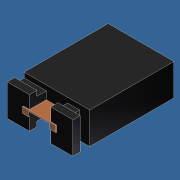
# Autodesk Inventor part: 2009_CTS_CopperPost2
Saved by Autodesk Inventor 2012 (Build 160160000, 160)
## iProperties
Company: Team 801
Created: 2009-01-31
Part Number: 2009_CTS_CopperPost2
Document SubType Name: Modeling
Designer: Jeffrey M
Density: 1 g/cm^3
Material: Default
Title: 2009_CTS_CopperPost2
Author: Jeffrey M
Autodesk Inventor part; units mm, degrees
ref_plane "YZ Plane" through (0, 0, 0) normal (1, 0, 0) x (0, 1, 0)
ref_plane "XZ Plane" through (0, 0, 0) normal (0, 1, 0) x (-1, 0, 0)
ref_plane "XY Plane" through (0, 0, 0) normal (0, 0, 1) x (1, 0, 0)
sketch "Sketch1" plane through (0, 0, 0) normal (0, 0, 1) x (1, 0, 0)
  line L0 (-37.8857, 18.2857) -> (-32.9327, 18.2857)
  line L1 (-32.9327, 18.2857) -> (-32.9327, 15.8981)
  line L2 (-32.9327, 15.8981) -> (-37.8857, 15.8981)
  line L3 (-37.8857, 15.8981) -> (-37.8857, 18.2857)
  dimension "d0" = 4.953
  dimension "d1" = 2.3876
  constraints: 8 end point, 2 parallel, 1 horizontal, 1 perpendicular
  measures "d0" distance of L0.start L0.end
  measures "d1" distance of L0.end L1.end
extrude "Extrusion1" add sketch "Sketch1" along normal blind 7.62
sketch "Sketch2" plane through (-37.8857, 15.8981, 0) normal (0, -1, 0) x (1, 0, 0)
  line L0 (4.953, 7.62) -> (0, 7.62) projected
  line L1 (1.6764, 7.62) -> (3.2766, 7.62)
  line L2 (3.2766, 7.62) -> (3.2766, 6.35)
  line L3 (3.2766, 6.35) -> (1.6764, 6.35)
  line L4 (1.6764, 6.35) -> (1.6764, 7.62)
  line L5 (0, 0) -> (0, 7.62) projected
  line L6 (4.953, 0) -> (4.953, 7.62) projected
  line L7 (4.953, 7.0612) -> (4.191, 7.0612)
  line L8 (4.191, 7.0612) -> (4.191, 6.35)
  line L9 (4.191, 6.35) -> (4.953, 6.35)
  line L10 (4.953, 6.35) -> (4.953, 7.0612)
  line L11 (0, 12.9286) -> (0.762, 12.9286)
  line L12 (0.762, 12.9286) -> (0.762, 12.2174)
  line L13 (0.762, 12.2174) -> (0, 12.2174)
  line L14 (0, 12.2174) -> (0, 12.9286)
  dimension "d4" = 1.6764
  dimension "d5" = 1.6764
  dimension "d6" = 1.27
  dimension "d9" = 0.5588
  dimension "d12" = 0
  dimension "d13" = 0.762
  dimension "d14" = 0.762
  constraints: 24 end point, 6 parallel, 3 horizontal, 3 perpendicular, 3 point on line
  measures "d4" distance of L0.start L1.end
  measures "d5" distance of L0.end L1.start
  measures "d6" distance of L1.end L2.end
  measures "d9" distance of L0.start L7.start
  measures "d12" distance between parallel lines of L3 L9
  measures "d13" distance of L7.start L7.end
  measures "d14" distance of L11.start L11.end
extrude "Extrusion2" cut sketch "Sketch2" against normal blind 13.4874
sketch "Sketch3" plane through (-33.6947, 15.8981, 7.0612) normal (1, 0, 0) x (0, 0, -1)
  line L0 (0, 2.3876) -> (0.7112, 2.3876) projected
  line L1 (0.7112, 0) -> (0, 0) projected
  line L2 (0.7112, 0) -> (0.7112, 2.3876) projected
  line L3 (0, 2.3876) -> (0.7112, 2.3876)
  line L4 (0.7112, 2.3876) -> (0.7112, 2.0066)
  line L5 (0.7112, 2.0066) -> (0, 2.0066)
  line L6 (0, 2.0066) -> (0, 2.3876)
  line L7 (0, 0) -> (0.7112, 0)
  line L8 (0.7112, 0) -> (0.7112, 0.381)
  line L9 (0.7112, 0.381) -> (0, 0.381)
  line L10 (0, 0.381) -> (0, 0)
  dimension "d15" = 0.381
  dimension "d16" = 0.381
  constraints: 16 end point, 4 parallel, 2 horizontal, 2 perpendicular, 2 point on line
  measures "d15" distance between parallel lines of L0 L5
  measures "d16" distance between parallel lines of L1 L9
extrude "Extrusion3" cut sketch "Sketch3" against normal blind 13.4874
sketch "Sketch4" plane through (0, 0, 7.62) normal (0, 0, 1) x (1, 0, 0)
  line L0 (-36.2093, 15.8981) -> (-36.2093, 18.2857) projected
  line L1 (-37.8857, 18.2857) -> (-36.2093, 18.2857) projected
  line L2 (-36.2093, 15.8981) -> (-37.8857, 15.8981) projected
  line L3 (-36.2093, 17.3205) -> (-36.6665, 17.3205)
  line L4 (-36.6665, 17.3205) -> (-36.6665, 16.8633)
  line L5 (-36.6665, 16.8633) -> (-36.2093, 16.8633)
  line L6 (-36.2093, 16.8633) -> (-36.2093, 17.3205)
  line L7 (-34.6091, 18.2857) -> (-34.6091, 15.8981) projected
  line L8 (-32.9327, 15.8981) -> (-34.6091, 15.8981) projected
  line L9 (-32.9327, 18.2857) -> (-32.9327, 15.8981) projected
  line L10 (-34.6091, 18.2857) -> (-32.9327, 18.2857) projected
  line L11 (-34.6091, 17.3205) -> (-34.1519, 17.3205)
  line L12 (-34.1519, 17.3205) -> (-34.1519, 16.8633)
  line L13 (-34.1519, 16.8633) -> (-34.6091, 16.8633)
  line L14 (-34.6091, 16.8633) -> (-34.6091, 17.3205)
  dimension "d19" = 0.4572
  dimension "d20" = 0.4572
  dimension "d21" = 0.4572
  dimension "d22" = 0.4572
  dimension "d23" = 0.9652
  dimension "d24" = 0.9652
  dimension "d25" = 0.9652
  constraints: 16 end point, 4 parallel, 2 horizontal, 2 perpendicular, 2 point on line
  measures "d19" distance of L3.start L3.end
  measures "d20" distance of L11.start L11.end
  measures "d21" distance of L11.end L12.end
  measures "d22" distance of L3.end L4.end
  measures "d23" distance between parallel lines of L1 L3
  measures "d24" distance between parallel lines of L10 L11
  measures "d25" distance between parallel lines of L5 L2
extrude "Extrusion4" add sketch "Sketch4" against normal mid plane 0.127 contours L5 L4 L3 L0 | L11 L12 L13 L7
sketch "Sketch5" plane through (-37.8857, 15.8981, 6.35) normal (0, 0, 1) x (1, 0, 0)
  line L0 (3.2766, 0.381) -> (3.2766, 2.0066) projected
  line L1 (1.6764, 1.4224) -> (1.6764, 0.9652) projected
  line L2 (1.2192, 1.4224) -> (1.6764, 1.4224) projected
  line L3 (1.2192, 0.9652) -> (1.2192, 1.4224) projected
  line L4 (1.6764, 0.9652) -> (1.2192, 0.9652) projected
  line L5 (3.2766, 1.4224) -> (3.7338, 1.4224) projected
  line L6 (3.2766, 0.9652) -> (3.2766, 1.4224) projected
  line L7 (3.7338, 0.9652) -> (3.2766, 0.9652) projected
  line L8 (3.7338, 1.4224) -> (3.7338, 0.9652) projected
  line L9 (1.6764, 1.4224) -> (3.2766, 1.4224)
  line L10 (3.2766, 1.4224) -> (3.2766, 1.3261)
  line L11 (3.2766, 1.3261) -> (1.6764, 1.3261)
  line L12 (1.6764, 1.3261) -> (1.6764, 1.4224)
  constraints: 8 end point, 2 parallel, 1 horizontal, 1 perpendicular, 1 point on line
extrude "Extrusion5" add sketch "Sketch5" along normal blind 1.3335 contours L11 L1 L9 L0
equation "\"d5\" = d4"
equation "\"d14\" = d13"
equation "\"d16\" = d15"
equation "\"d20\" = d19"
equation "\"d21\" = d20"
equation "\"d22\" = d21"
equation "\"d24\" = d23"
body "Solid1"
